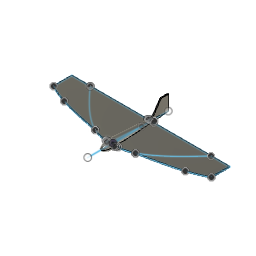
Glider plane v4 (Autodesk Fusion 360 design; units mm, degrees)
Autodesk Fusion 360 part; units mm, degrees
note: some values were not read from the file. Set by a fixed rule: which sketch regions a step uses.
sketch "Sketch1" plane through (0, 0, 0) normal (0, 1, 0) x (1, 0, 0)
sketch "Sketch2" plane through (0, 0, 0) normal (0, 0, 1) x (1, 0, 0)
  line L0 (-0.0319, -25) -> (-0.0319, 105)
  line L1 (-0.0319, 4.8019) -> (8.1294, 4.8019)
  spline S0 degree 5 poles (-0.0319, -25) (0.4387, -24.7877) (1.3377, -24.3149) (2.5595, -23.461) (3.9347, -22.0325) (5.2413, -19.7847) (6.176, -17.1497) (6.8216, -14.275) (7.2723, -11.295) (7.6093, -8.2635) (7.8701, -5.0621) (8.0567, -1.456) (8.1523, 2.821) (8.1331, 7.998) (7.9854, 14.1759) (7.7078, 21.3207) (7.3079, 29.2997) (6.8002, 37.9038) (6.2041, 46.8737) (5.5416, 55.9235) (4.8355, 64.7652) (4.1072, 73.1326) (3.3749, 80.8047) (2.6513, 87.6324) (1.9446, 93.5245) (1.2596, 98.4336) (0.7307, 101.5603) (0.3451, 103.4549) (0.0929, 104.5182) (-0.0319, 105) knots 0 0 0 0 0 0 0.04 0.08 0.12 0.16 0.2 0.24 0.28 0.32 0.36 0.4 0.44 0.48 0.52 0.56 0.6 0.64 0.68 0.72 0.76 0.8 0.84 0.88 0.92 0.96 1 1 1 1 1 1
  point P0 (5, -20)
  point P1 (7.3102, -10.7636)
  point P2 (4.0647, 73.4133)
  dimension "d1" = 130
  constraint vertical L0
  constraint coincident L0 L1.start
  constraint perpendicular L0 L1
  measures "d1" distance of L0.start L0.end
revolve "Revolve1" add sketch "Sketch2" angle 360 about axis through (-0.0319, -25, 0) along (0, 1, 0)
sketch "Sketch3" plane through (0, 0, 0) normal (1, 0, 0) x (0, 1, 0)
  spline S0 degree 5 poles (-3, 0) (-3.0505, 0.2431) (-3.0079, 0.7013) (-2.5131, 1.3049) (-0.9783, 1.9395) (2.4326, 2.4428) (7.2539, 2.6719) (13.3247, 2.6582) (20.4655, 2.4364) (28.5063, 2.0397) (37.3088, 1.495) (44.8819, 0.956) (50.836, 0.4984) (54.9254, 0.17) (57, 0) knots 0 0 0 0 0 0 0.1 0.2 0.3 0.4 0.5 0.6 0.7 0.8 0.9 1 1 1 1 1 1
  spline S1 degree 5 poles (-3, 0) (-2.9668, -0.1175) (-2.7678, -0.3391) (-2.0717, -0.6315) (-0.3362, -0.94) (3.2156, -1.1865) (8.0871, -1.3001) (14.1339, -1.2954) (21.1921, -1.1889) (29.1039, -0.9964) (37.74, -0.731) (45.1548, -0.4677) (50.9774, -0.2439) (54.9734, -0.0832) (57, 0) knots 0 0 0 0 0 0 0.1 0.2 0.3 0.4 0.5 0.6 0.7 0.8 0.9 1 1 1 1 1 1
  point P0 (0, 2)
  point P1 (1, -1)
sketch "Sketch4" plane through (0, 0, 0) normal (0, 0, 1) x (1, 0, 0)
sketch "Sketch5" plane through (0, 0, 0) normal (0, 0, 1) x (1, 0, 0)
  spline S0 degree 5 poles (0, 0) (1.8898, -0.5282) (5.7193, -1.3867) (11.6129, -2.0803) (19.7749, -1.7971) (30.5113, 0.6796) (41.8103, 5.3928) (53.6773, 12.3639) (66.073, 21.4372) (78.9433, 32.397) (92.2334, 45.0258) (103.1664, 56.325) (111.5231, 65.4237) (117.1629, 71.7624) (120, 75) knots 0 0 0 0 0 0 0.1 0.2 0.3 0.4 0.5 0.6 0.7 0.8 0.9 1 1 1 1 1 1
  line L0 (120, 75) -> (0, 75)
  line L1 (0, 75) -> (0, 0)
  spline S1 degree 5 poles (12.3687, -1.7473) (12.2185, -1.7817) (11.9224, -1.8524) (11.4909, -1.9647) (10.9414, -2.1268) (10.3009, -2.3516) (9.7112, -2.601) (9.1773, -2.8771) (8.7033, -3.182) (8.289, -3.5157) (7.9307, -3.8762) (7.6858, -4.1847) (7.524, -4.4266) (7.4258, -4.5925) (7.3791, -4.6766) knots 0 0 0 0 0 0 0.1 0.2 0.3 0.4 0.5 0.6 0.7 0.8 0.9 1 1 1 1 1 1
  line L2 (7.3791, -4.6766) -> (7.3791, -1.4402)
  spline S2 degree 5 poles (6.3288, 75) (6.2715, 75.0209) (6.156, 75.0683) (5.9802, 75.1559) (5.7405, 75.3061) (5.4316, 75.5531) (5.1128, 75.8634) (4.7836, 76.2401) (4.4442, 76.6817) (4.0955, 77.1827) (3.7383, 77.7374) (3.4465, 78.22) (3.2245, 78.6022) (3.0751, 78.8659) (3, 79) knots 0 0 0 0 0 0 0.1 0.2 0.3 0.4 0.5 0.6 0.7 0.8 0.9 1 1 1 1 1 1
  line L3 (3, 79) -> (3, 75)
  line L4 (0, 110) -> (0, -50)
  line L5 (-3, 79) -> (-3, 75)
  spline S3 degree 5 poles (-6.3288, 75) (-6.2715, 75.0209) (-6.156, 75.0683) (-5.9802, 75.1559) (-5.7405, 75.3061) (-5.4316, 75.5531) (-5.1128, 75.8634) (-4.7836, 76.2401) (-4.4442, 76.6817) (-4.0955, 77.1827) (-3.7383, 77.7374) (-3.4465, 78.22) (-3.2245, 78.6022) (-3.0751, 78.8659) (-3, 79) knots 0 0 0 0 0 0 0.1 0.2 0.3 0.4 0.5 0.6 0.7 0.8 0.9 1 1 1 1 1 1
  line L6 (6.7478, 74.8468) -> (5.9098, 75.1532)
  line L7 (3.3369, 78.3981) -> (2.6631, 79.6019)
  line L8 (-6.7478, 74.8468) -> (-5.9098, 75.1532)
  line L9 (-3.3369, 78.3981) -> (-2.6631, 79.6019)
  line L10 (-120, 75) -> (0, 75)
  spline S4 degree 5 poles (0, 0) (-1.8898, -0.5282) (-5.7193, -1.3867) (-11.6129, -2.0803) (-19.7749, -1.7971) (-30.5113, 0.6796) (-41.8103, 5.3928) (-53.6773, 12.3639) (-66.073, 21.4372) (-78.9433, 32.397) (-92.2334, 45.0258) (-103.1664, 56.325) (-111.5231, 65.4237) (-117.1629, 71.7624) (-120, 75) knots 0 0 0 0 0 0 0.1 0.2 0.3 0.4 0.5 0.6 0.7 0.8 0.9 1 1 1 1 1 1
  line L11 (-14.0277, 3.921) -> (14.0277, -3.921)
  line L12 (106.6974, 59.8194) -> (133.3026, 90.1806)
  line L13 (14.0277, 3.921) -> (-14.0277, -3.921)
  line L14 (-106.6974, 59.8194) -> (-133.3026, 90.1806)
  spline S5 degree 5 poles (-12.3687, -1.7473) (-12.2185, -1.7817) (-11.9224, -1.8524) (-11.4909, -1.9647) (-10.9414, -2.1268) (-10.3009, -2.3516) (-9.7112, -2.601) (-9.1773, -2.8771) (-8.7033, -3.182) (-8.289, -3.5157) (-7.9307, -3.8762) (-7.6858, -4.1847) (-7.524, -4.4266) (-7.4258, -4.5925) (-7.3791, -4.6766) knots 0 0 0 0 0 0 0.1 0.2 0.3 0.4 0.5 0.6 0.7 0.8 0.9 1 1 1 1 1 1
  line L15 (13.0969, -1.5807) -> (11.6405, -1.9139)
  line L16 (7.6738, -4.1459) -> (7.0845, -5.2073)
  line L17 (-13.0969, -1.5807) -> (-11.6405, -1.9139)
  line L18 (-7.6738, -4.1459) -> (-7.0845, -5.2073)
  line L19 (-7.3791, -4.6766) -> (-7.3791, -1.4402)
  spline S6 degree 5 poles (40, 5) (43.1814, 5.5793) (49.4761, 6.7463) (58.7136, 8.5216) (70.6144, 10.9391) (84.7448, 14.0516) (98.0471, 17.2646) (110.4226, 20.5901) (121.7779, 24.0395) (132.0631, 27.6188) (141.3122, 31.324) (147.9311, 34.3828) (152.4806, 36.7273) (155.3322, 38.3124) (156.7127, 39.1104) knots 0 0 0 0 0 0 0.1 0.2 0.3 0.4 0.5 0.6 0.7 0.8 0.9 1 1 1 1 1 1
  line L20 (120, 75) -> (156.7127, 75)
  line L21 (156.7127, 39.1104) -> (156.7127, 75)
  spline S7 degree 5 poles (-40, 5) (-43.1814, 5.5793) (-49.4761, 6.7463) (-58.7136, 8.5216) (-70.6144, 10.9391) (-84.7448, 14.0516) (-98.0471, 17.2646) (-110.4226, 20.5901) (-121.7779, 24.0395) (-132.0631, 27.6188) (-141.3122, 31.324) (-147.9311, 34.3828) (-152.4806, 36.7273) (-155.3322, 38.3124) (-156.7127, 39.1104) knots 0 0 0 0 0 0 0.1 0.2 0.3 0.4 0.5 0.6 0.7 0.8 0.9 1 1 1 1 1 1
  line L22 (25.6009, 2.3779) -> (54.3991, 7.6221)
  line L23 (147.6469, 33.8698) -> (165.7786, 44.3509)
  line L24 (-25.6009, 2.3779) -> (-54.3991, 7.6221)
  line L25 (-147.6469, 33.8698) -> (-165.7786, 44.3509)
  line L26 (-156.7127, 39.1104) -> (-156.7127, 75)
  line L27 (-120, 75) -> (-156.7127, 75)
  point P0 (40, 5)
  point P1 (9, -3)
  point P2 (5, 76)
  point P3 (-5, 76)
  point P4 (-40, 5)
  point P5 (-9, -3)
  point P6 (120.3507, 23.6977)
  point P7 (-120.3507, 23.6977)
  dimension "d9" = 90
  constraint coincident S0.start L1.end
  constraint horizontal L0
  constraint perpendicular L0 L1
  constraint coincident S0 S1.start
  constraint coincident S0 L2.end
  constraint vertical L2
  constraint coincident L0 S2.start
  constraint coincident L0 L3.end
  constraint perpendicular L0 L3
  constraint vertical L4
  constraint midpoint S2.start L6
  constraint midpoint S2.end L7
  constraint midpoint S0.start L11
  constraint midpoint S0.end L12
  constraint midpoint S1.start L15
  constraint midpoint S1.end L16
  constraint symmetric S0.start L4 L1.end
  constraint symmetric P0 L4 P4
  constraint symmetric S0.end L4 L10.start
  constraint symmetric L0.end L4 L1.start
  constraint symmetric S1.start L4 S5.start
  constraint symmetric P1 L4 P5
  constraint symmetric S1.end L4 S5.end
  constraint symmetric L2.end L4 L19.end
  constraint symmetric S2.start L4 S3.start
  constraint symmetric P2 L4 P3
  constraint symmetric S2.end L4 L5.start
  constraint symmetric L3.end L4 L5.end
  constraint symmetric L4 L6.start L8.start
  constraint symmetric L4 L6.end L8.end
  constraint symmetric L4 L7.start L9.start
  constraint symmetric L4 L7.end L9.end
  constraint symmetric L4 L11.start L13.start
  constraint symmetric L4 L11.end L13.end
  constraint symmetric L4 L12.start L14.start
  constraint symmetric L4 L12.end L14.end
  constraint symmetric L4 L15.start L17.start
  constraint symmetric L4 L15.end L17.end
  constraint symmetric L4 L16.start L18.start
  constraint symmetric L4 L16.end L18.end
  constraint coincident P0 S6.start
  constraint parallel L0 L20
  constraint midpoint P0 L22
  constraint midpoint S6.end L23
  constraint symmetric S0.end L1 L10.start
  constraint symmetric L1 P0 P4
  constraint symmetric L1 P6 P7
  constraint symmetric L1 S6.end S7.end
  constraint symmetric L1 L20.end L26.end
  constraint symmetric L1 L22.start L24.start
  constraint symmetric L1 L22.end L24.end
  constraint symmetric L1 L23.start L25.start
  constraint symmetric L1 L23.end L25.end
  measures "d9" angle of L20 L21
extrude "Extrude3" add sketch "Sketch5" along normal mid plane 2 contours S0 L0 L1 L4 | L1 L4 L10 S4 | S0 S1 L2 L11 | S4 L13 S5 L19 | S1 L2 L11 | L13 S5 L19 | L0 S2 L3 | L5 S3 L10 | S0 S6 L20 L21 | S4 S7 L26 L27
sketch "Sketch7" plane through (0, 0, 0) normal (1, 0, 0) x (0, 1, 0)
  line L0 (75, 0) -> (95, 30)
  line L1 (95, 30) -> (110, 30)
  line L2 (110, 30) -> (110, 15)
  line L3 (110, 15) -> (110, 0)
  line L4 (110, 0) -> (75, 0)
  spline S0 degree 5 poles (81.5915, 9.8872) (81.4243, 9.6832) (81.0828, 9.2821) (80.5489, 8.7007) (79.7932, 7.9669) (78.7707, 7.1233) (77.6638, 6.3592) (76.4665, 5.6803) (75.1774, 5.0882) (73.8016, 4.5778) (72.3465, 4.1422) (71.1245, 3.8484) (70.1776, 3.6567) (69.533, 3.5415) (69.2074, 3.487) knots 0 0 0 0 0 0 0.1 0.2 0.3 0.4 0.5 0.6 0.7 0.8 0.9 1 1 1 1 1 1
  line L5 (69.2074, 3.487) -> (76.4436, 2.1654)
  point P0 (76.7449, 5.86)
  constraint horizontal L1
  constraint perpendicular L1 L2
  constraint perpendicular L1 L3
  constraint perpendicular L3 L4
  constraint coincident L0 S0.start
  constraint coincident L0 L5.end
extrude "Extrude4" add sketch "Sketch7" along normal mid plane 2
